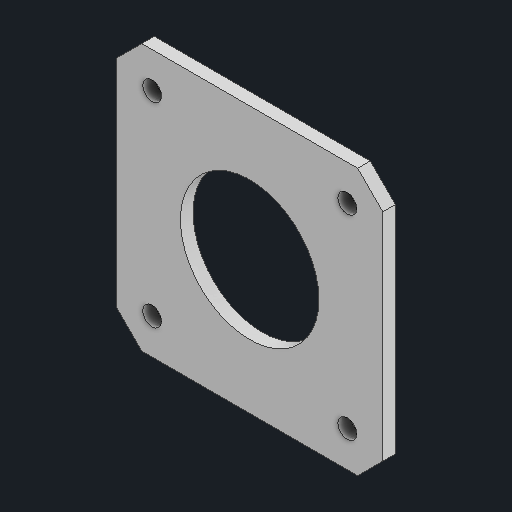
# Autodesk Inventor part: Stepper_spacer
Saved by Autodesk Inventor 2026.1 (Build 301233020, 233B)
## iProperties
Created: 2026-03-04
Part Number: Stepper_spacer
Material: Generic
Document SubType Name: Modeling
Designer: Mikke
Density: 1 g/cm^3
Appearance: Default
Author: Mikke
Autodesk Inventor part; units mm, degrees
ref_plane "YZ Plane" through (0, 0, 0) normal (1, 0, 0) x (0, 1, 0)
ref_plane "XZ Plane" through (0, 0, 0) normal (0, 1, 0) x (-1, 0, 0)
ref_plane "XY Plane" through (0, 0, 0) normal (0, 0, 1) x (1, 0, 0)
sketch "Sketch1" plane through (0, 0, 0) normal (0, 0, 1) x (1, 0, 0)
  circle A0 centre (0, 51.9685) radius 11 projected
  line L0 (21.15, 34.8185) -> (21.15, 69.1185) projected
  line L1 (21.15, 69.1185) -> (17.15, 73.1185) projected
  line L2 (17.15, 73.1185) -> (-17.15, 73.1185) projected
  line L3 (-17.15, 73.1185) -> (-21.15, 69.1185) projected
  line L4 (-21.15, 69.1185) -> (-21.15, 34.8185) projected
  line L5 (-21.15, 34.8185) -> (-17.15, 30.8185) projected
  line L6 (-17.15, 30.8185) -> (17.15, 30.8185) projected
  line L7 (17.15, 30.8185) -> (21.15, 34.8185) projected
  circle A1 centre (-15.5, 36.4685) radius 1.5 projected
  circle A2 centre (15.5, 36.4685) radius 1.5 projected
  circle A3 centre (15.5, 67.4685) radius 1.5 projected
  circle A4 centre (-15.5, 67.4685) radius 1.5 projected
  point P0 (0, 0)
extrude "Extrusion1" add sketch "Sketch1" along normal blind 2
body "Solid1"
